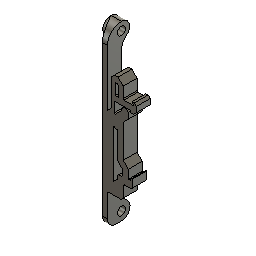
manta_m8p_v2_0_din_clip_back (Autodesk Fusion 360 design; units mm, degrees)
Autodesk Fusion 360 part; units mm, degrees
sketch "Sketch1" plane through (0, 0, 0) normal (0, 0, 1) x (1, 0, 0)
  line L0 (0, 0) -> (0, 42.5)
  line L1 (0, 42.5) -> (2, 44.5)
  line L2 (2, 44.5) -> (2, 60)
  line L3 (2, 60) -> (4, 62)
  line L4 (4, 62) -> (6, 62)
  line L5 (6, 62) -> (9, 59)
  line L6 (9, 59) -> (9, 52.75)
  line L7 (9, 52.75) -> (9.5, 52.25)
  line L8 (9.5, 52.25) -> (14.77, 52.25)
  line L9 (14.77, 52.25) -> (15.01, 52.49)
  line L10 (15.01, 52.49) -> (14.1, 53.4)
  line L11 (14.1, 53.4) -> (14.1, 53.8)
  line L12 (14.1, 53.8) -> (15.4, 53.8)
  line L13 (15.4, 53.8) -> (16.6, 52.6)
  line L14 (16.6, 52.6) -> (16.6, 49.5)
  line L15 (16.6, 49.5) -> (15.05, 47.95)
  line L16 (15.05, 47.95) -> (13.45, 47.95)
  line L17 (13.1, 48.3) -> (13.1, 49)
  line L18 (13.1, 49) -> (4.25, 49)
  line L19 (3.75, 48.5) -> (3.75, 43.025)
  line L20 (4.4748, 42.7248) -> (8.25, 46.5)
  line L21 (8.25, 46.5) -> (8.25, 47.5)
  line L22 (8.25, 47.5) -> (9.25, 48.5)
  line L23 (9.25, 48.5) -> (11.025, 48.5)
  line L24 (11.025, 48.5) -> (12.025, 47.5)
  line L25 (12.025, 47.5) -> (12.025, 44)
  line L26 (12.025, 44) -> (9, 40.975)
  line L27 (9, 40.975) -> (9, 21.975)
  line L28 (9, 21.975) -> (12, 18.975)
  line L29 (12, 18.975) -> (12, 13.975)
  line L30 (12, 13.975) -> (13.1, 13.975)
  line L31 (13.1, 13.975) -> (13.1, 14.475)
  line L32 (13.1, 14.475) -> (14.1, 15.475)
  line L33 (14.1, 15.475) -> (14.6, 15.475)
  line L34 (14.6, 15.475) -> (14.6, 10.975)
  line L35 (14.6, 10.975) -> (13.6, 9.975)
  line L36 (13.6, 9.975) -> (9.5, 9.975)
  line L37 (9.5, 9.975) -> (9, 9.475)
  line L38 (9, 9.475) -> (9, 3)
  line L39 (9, 3) -> (6, 0)
  line L40 (6, 0) -> (0, 0)
  line L41 (13.45, 47.95) -> (13.1, 48.3)
  line L42 (3.75, 48.5) -> (4.25, 49)
  line L43 (4.4748, 42.7248) -> (3.75, 43.025)
  line L44 (3.5, 8.7034) -> (3.5, 36.3034)
  line L45 (3.5, 36.3034) -> (5.5, 35.475)
  line L46 (5.5, 35.475) -> (5.5, 20.475)
  line L47 (5.5, 20.475) -> (8.5, 17.475)
  line L48 (8.5, 17.475) -> (8.5, 13.975)
  line L49 (8.5, 13.975) -> (8, 13.475)
  line L50 (8, 13.475) -> (6.5, 13.475)
  line L51 (6.5, 13.475) -> (5.5, 12.475)
  line L52 (5.5, 12.475) -> (5.5, 10.7034)
  line L53 (5.5, 10.7034) -> (3.5, 8.7034)
  line L54 (4.5, 52) -> (6.5, 52)
  line L55 (6.5, 52) -> (6.5, 57.5)
  line L56 (6.5, 57.5) -> (5.5, 58.5)
  line L57 (5.5, 58.5) -> (4.5, 58.5)
  line L58 (4.5, 58.5) -> (4.5, 52)
  dimension "d1" = 42.5
  dimension "d2" = 135
  dimension "d3" = 2
  dimension "d4" = 62
  dimension "d5" = 7
  dimension "d6" = 135
  dimension "d7" = 9.75
  dimension "d8" = 6.25
  dimension "d9" = 5.27
  dimension "d10" = 5.1
  dimension "d11" = 1.55
  dimension "d12" = 2
  dimension "d13" = 0.4
  dimension "d14" = 2
  dimension "d15" = 135
  dimension "d16" = 7.6
  dimension "d17" = 3.1
  dimension "d18" = 5.85
  dimension "d19" = 3.5
  dimension "d20" = 1.6
  dimension "d21" = 135
  dimension "d22" = 0.7
  dimension "d23" = 3.25
  dimension "d24" = 1.75
  dimension "d25" = 135
  dimension "d26" = 0.5
  dimension "d27" = 45
  dimension "d28" = 112.5
  dimension "d29" = 5.475
  dimension "d30" = 4.5
  dimension "d31" = 0.5
  dimension "d32" = 3.775
  dimension "d33" = 1
  dimension "d34" = 1
  dimension "d35" = 1
  dimension "d36" = 135
  dimension "d37" = 135
  dimension "d39" = 9
  dimension "d40" = 3.5
  dimension "d41" = 19
  dimension "d42" = 3
  dimension "d43" = 5
  dimension "d44" = 1.1
  dimension "d45" = 135
  dimension "d46" = 0.5
  dimension "d47" = 1.5
  dimension "d48" = 0.5
  dimension "d49" = 5.5
  dimension "d50" = 135
  dimension "d51" = 1
  dimension "d52" = 5.6
  dimension "d53" = 135
  dimension "d54" = 0.5
  dimension "d55" = 6
  dimension "d56" = 2
  dimension "d57" = 6.5
  dimension "d58" = 135
  dimension "d59" = 1
  dimension "d60" = 2.5
  dimension "d61" = 3.5
  dimension "d62" = 3.5
  dimension "d63" = 2
  dimension "d64" = 112.5
  dimension "d65" = 135
  dimension "d66" = 5
  dimension "d67" = 0.5
  dimension "d68" = 1.5
  dimension "d69" = 2
  dimension "d70" = 135
  dimension "d71" = 27.6
  dimension "d72" = 3.5
  dimension "d73" = 15
  dimension "d74" = 135
  dimension "d75" = 3.5
  constraint coincident L0.start L40.end
  constraint vertical L0
  constraint parallel L0 L2
  constraint parallel L1 L3
  constraint horizontal L4
  constraint perpendicular L4 L6
  constraint perpendicular L3 L7
  constraint perpendicular L5 L9
  constraint vertical L11
  constraint perpendicular L11 L12
  constraint parallel L11 L14
  constraint perpendicular L10 L15
  constraint perpendicular L14 L16
  constraint perpendicular L16 L17
  constraint perpendicular L17 L18
  constraint perpendicular L18 L19
  constraint parallel L19 L21
  constraint perpendicular L19 L23
  constraint perpendicular L23 L25
  constraint parallel L25 L27
  constraint perpendicular L26 L28
  constraint parallel L27 L29
  constraint perpendicular L29 L30
  constraint perpendicular L30 L31
  constraint perpendicular L31 L33
  constraint perpendicular L33 L34
  constraint perpendicular L34 L36
  constraint perpendicular L36 L38
  constraint parallel L37 L39
  constraint perpendicular L38 L40
  constraint horizontal L8
  constraint perpendicular L9 L10
  constraint parallel L20 L26
  constraint parallel L38 L44
  constraint parallel L44 L46
  constraint parallel L46 L48
  constraint perpendicular L46 L50
  constraint parallel L49 L51
  constraint perpendicular L50 L52
  constraint perpendicular L19 L54
  constraint perpendicular L54 L55
  constraint perpendicular L55 L57
  constraint parallel L55 L58
  measures "d1" distance of L0.start L0.end
  measures "d2" angle of L0 L1
  measures "d3" distance of L0 L2
  measures "d4" distance of L4 L40
  measures "d5" distance of L2 L6
  measures "d6" angle of L5 L6
  measures "d7" distance of L4 L8
  measures "d8" distance of L5.end L6.end
  measures "d9" distance of L7.end L8.end
  measures "d10" distance of L6 L11
  measures "d11" distance of L8 L12
  measures "d12" distance of L3.end L4.end
  measures "d13" distance of L10.end L11.end
  measures "d14" distance of L2 L3.end
  measures "d15" angle of L12 L13
  measures "d16" distance of L6 L14
  measures "d17" distance of L13.end L14.end
  measures "d18" distance of L12 L16
  measures "d19" distance of L14 L17
  measures "d20" distance of L15.end L16.end
  measures "d21" angle of L16 L41
  measures "d22" distance of L17.end L17.start
  measures "d23" distance of L8 L18
  measures "d24" distance of L2 L19
  measures "d25" angle of L18 L42
  measures "d26" distance of L19 L18.end
  measures "d27" angle of L19 L20
  measures "d28" angle of L20 L43
  measures "d29" distance of L19.end L19.start
  measures "d30" distance of L19 L21
  measures "d31" distance of L18 L23
  measures "d32" distance of L21 L25
  measures "d33" distance of L20.end L21.end
  measures "d34" distance of L23.end L25
  measures "d35" distance of L21 L22.end
  measures "d36" angle of L21 L22
  measures "d37" angle of L24 L25
  measures "d39" distance of L0 L27
  measures "d40" distance of L24.end L25.end
  measures "d41" distance of L26.end L27.end
  measures "d42" distance of L27 L29
  measures "d43" distance of L28.end L29.end
  measures "d44" distance of L29.end L30.end
  measures "d45" angle of L31 L32
  measures "d46" distance of L30.end L31.end
  measures "d47" distance of L31 L34
  measures "d48" distance of L32.end L33.end
  measures "d49" distance of L33 L36
  measures "d50" angle of L34 L35
  measures "d51" distance of L34 L35.end
  measures "d52" distance of L34 L38
  measures "d53" angle of L37 L38
  measures "d54" distance of L36.end L38
  measures "d55" distance of L39.end L0.start
  measures "d56" distance of L54.start L54.end
  measures "d57" distance of L54 L57
  measures "d58" angle of L56 L57
  measures "d59" distance of L56.end L57.end
  measures "d60" distance of L2 L58
  measures "d61" distance of L4 L57
  measures "d62" distance of L0 L44
  measures "d63" distance of L44 L46
  measures "d64" angle of L45 L46
  measures "d65" angle of L46 L47
  measures "d66" distance of L44 L48
  measures "d67" distance of L48 L49.end
  measures "d68" distance of L49.end L50.end
  measures "d69" distance of L44 L52
  measures "d70" angle of L48 L49
  measures "d71" distance of L44.start L44.end
  measures "d72" distance of L36 L50
  measures "d73" distance of L45.end L46.end
  measures "d74" angle of L52 L53
  measures "d75" distance of L47.end L48.end
extrude "Extrude1" add sketch "Sketch1" along normal blind 8
chamfer "Chamfer1" distance 1.8 angle 45 2 edges at (3, 0, 8) (3, 0, 0)
sketch "Sketch2" plane through (0, 0, 0) normal (-1, 0, 0) x (0, 0, 1)
  line L0 (8, 42.5) -> (0, 42.5)
  line L1 (-11.6951, 31.4875) -> (67.4923, 31.4875) construction
  line L2 (8, 74.8575) -> (8, -11.8825)
  line L3 (0, 49) -> (8, 49)
  line L4 (0, 13.975) -> (8, 13.975)
  circle A0 centre (0, 78.1175) radius 2.35
  circle A1 centre (0, -11.8825) radius 2.35
  line L5 (8, 82.8575) -> (-26.553, 82.8575) construction
  line L6 (8, -19.8825) -> (-15.8933, -19.8825) construction
  line L7 (0, 68.4445) -> (0, -1.8825)
  arc A2 (-3, -7.8825) -> (0, -1.8825) centre (-7.5, -1.8825) ccw
  arc A3 (0, 68.4445) -> (-2.9044, 74.3716) centre (-7.5, 68.4445) ccw
  arc A4 (8, 74.8575) -> (0, 82.8575) centre (0, 74.8575) ccw
  arc A5 (0, 82.8575) -> (-2.9044, 74.3716) centre (0, 78.1175) ccw
  line L8 (0, -16.8825) -> (3, -16.8825)
  arc A6 (3, -16.8825) -> (8, -11.8825) centre (3, -11.8825) ccw
  arc A7 (-3, -7.8825) -> (0, -16.8825) centre (0, -11.8825) ccw
  line L9 (0, 1.8) -> (1.8, 0)
  line L10 (1.8, 0) -> (6.2, 0)
  line L11 (6.2, 0) -> (8, 1.8)
  line L12 (8, 1.8) -> (8, 42.5)
  line L13 (0, 42.5) -> (0, 1.8)
  dimension "d80" = 102.74
  dimension "d81" = 4.7
  dimension "d82" = 46.63
  dimension "d83" = 43.37
  dimension "d84" = 8
  dimension "d85" = 15
  dimension "d86" = 15
  dimension "d89" = 10
  dimension "d90" = 5
  constraint vertical L2
  constraint symmetric L1 L5.start L6.start
  constraint symmetric L1 L3 L4
  constraint equal A0 A1
  constraint perpendicular L2 L5
  constraint perpendicular L2 L6
  constraint concentric A0 A5
  constraint tangent L5 A5
  constraint parallel L2 L7
  constraint tangent A3 A5
  constraint tangent L7 A3
  constraint tangent L7 A2
  constraint tangent A4 A5
  constraint tangent L2 A4
  constraint coincident L7 A4.centre
  constraint coincident L5 A4.end
  constraint concentric A1 A7
  constraint horizontal L8
  constraint tangent L8 A7
  constraint tangent L8 A6
  constraint tangent L2 A6
  constraint tangent A2 A7
  constraint coincident L7 A1.centre
  measures "d80" distance of L5.start L6.start
  measures "d81" diameter of A0
  measures "d82" distance of L1 A0.centre
  measures "d83" distance of L1 A1.centre
  measures "d84" distance of L2 A0.centre
  measures "d85" diameter of A3
  measures "d86" diameter of A2
  measures "d89" diameter of A7
  measures "d90" radius of A6
extrude "Extrude2" add sketch "Sketch2" along normal blind 3
sketch "Sketch3" plane through (-3, 0, 0) normal (-1, 0, 0) x (0, 0, 1)
  circle A0 centre (0, 78.1175) radius 2.35
  circle A1 centre (0, -11.8825) radius 2.35
  line L0 (0, 68.4445) -> (0, -1.8825)
  arc A2 (-3, -7.8825) -> (0, -1.8825) centre (-7.5, -1.8825) ccw
  arc A3 (-3, -7.8825) -> (0, -16.8825) centre (0, -11.8825) ccw
  line L1 (0, -16.8825) -> (3, -16.8825)
  arc A4 (3, -16.8825) -> (8, -11.8825) centre (3, -11.8825) ccw
  line L2 (8, -11.8825) -> (8, 74.8575)
  arc A5 (8, 74.8575) -> (0, 82.8575) centre (0, 74.8575) ccw
  arc A6 (0, 82.8575) -> (-2.9044, 74.3716) centre (0, 78.1175) ccw
  arc A7 (0, 68.4445) -> (-2.9044, 74.3716) centre (-7.5, 68.4445) ccw
  circle A8 centre (0, -11.8825) radius 5
  circle A9 centre (0, 78.1175) radius 4.74
  constraint concentric A1 A8
  constraint concentric A0 A9
extrude "Extrude3" add sketch "Sketch3" along normal blind 3 contours A6 A9 | A3 A8
fillet "Fillet1" radius 3 2 edges at (-3, 76.5826, 4.4846) (-3, -10.3014, 4.7434)
sketch "Sketch4" plane through (0, 0, 0) normal (0, 0, -1) x (-1, 0, 0)
  line L0 (0, 68.4445) -> (0, -1.8825)
  line L1 (0, -1.8825) -> (3, -1.8825)
  line L2 (3, -1.8825) -> (3, 68.4445)
  line L3 (3, 68.4445) -> (0, 68.4445)
  line L4 (-0.4, 1.8) -> (0, 1.8)
  line L5 (-0.4, 1.8) -> (-7.2343, 1.8)
  line L6 (0, 1.8) -> (0, 42.3343)
  line L7 (0, 42.3343) -> (-0.4, 42.3343)
  line L8 (-0.4, 42.3343) -> (-0.4, 1.8)
  point P0 (-0.4, 42.3343)
  constraint perpendicular L0 L4
  constraint collinear L4 L5
  constraint coincident L4.start L5.start
  constraint coincident L0 L4.end
  constraint coincident L0 L6.end
  constraint perpendicular L6 L7
  constraint coincident P0 L7.end
extrude "Extrude4" [suppressed]
